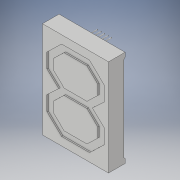
# Autodesk Inventor part: Digit
Saved by Autodesk Inventor 2019.3 (Build 233278000, 278)
## iProperties
Created: 2019-03-27
Part Number: Digit
Material: Generic
Document SubType Name: Modeling
Designer: Willist
Density: 1 g/cm^3
Appearance: Default
Author: Willist
Autodesk Inventor part; units mm, degrees
ref_plane "YZ Plane" through (0, 0, 0) normal (1, 0, 0) x (0, 1, 0)
ref_plane "XZ Plane" through (0, 0, 0) normal (0, 1, 0) x (-1, 0, 0)
ref_plane "XY Plane" through (0, 0, 0) normal (0, 0, 1) x (1, 0, 0)
sketch "Sketch1" plane through (0, 0, 0) normal (0, 0, 1) x (1, 0, 0)
  line L0 (-23.9, 34.85) -> (23.9, 34.85)
  line L1 (23.9, 34.85) -> (23.9, -34.85)
  line L2 (23.9, -34.85) -> (-23.9, -34.85)
  line L3 (-23.9, -34.85) -> (-23.9, 34.85)
  dimension "d0" = 47.8
  dimension "d1" = 69.7
  constraints: 8 end point, 2 parallel, 1 horizontal, 1 perpendicular
  measures "d0" distance of L1.end L2.end
  measures "d1" distance of L0.end L1.end
extrude "Extrusion1" add sketch "Sketch1" along normal blind 11
sketch "Sketch2" plane through (0, 0, 0) normal (0, 0, -1) x (-1, 0, 0)
  line L0 (-23.9, 34.85) -> (23.9, 34.85) projected
  line L1 (23.9, 34.85) -> (23.9, -34.85) projected
  line L2 (-23.9, 34.85) -> (23.9, 34.85)
  line L3 (23.9, 34.85) -> (23.9, 31.7132)
  line L4 (23.9, 31.7132) -> (-23.9, 31.7132)
  line L5 (-23.9, 31.7132) -> (-23.9, 34.85)
  line L6 (23.9, -34.85) -> (-23.9, -34.85) projected
  line L7 (-23.9, -34.85) -> (-23.9, 34.85) projected
  line L8 (23.9, -34.85) -> (-23.9, -34.85)
  line L9 (-23.9, -34.85) -> (-23.9, -31.7132)
  line L10 (-23.9, -31.7132) -> (23.9, -31.7132)
  line L11 (23.9, -31.7132) -> (23.9, -34.85)
  line L12 (-23.9, 34.85) -> (23.9, 34.85)
  line L13 (23.9, 34.85) -> (23.9, 31.7132)
  line L14 (23.9, 31.7132) -> (-23.9, 31.7132)
  line L15 (-23.9, 31.7132) -> (-23.9, 34.85)
  line L16 (-23.9, -31.7132) -> (23.9, -31.7132)
  line L17 (23.9, -31.7132) -> (23.9, -34.85)
  line L18 (23.9, -34.85) -> (-23.9, -34.85)
  line L19 (-23.9, -34.85) -> (-23.9, -31.7132)
  point P0 (0, 0)
  dimension "d4" = 3.1368
  dimension "d5" = 3.1368
  constraints: 32 end point, 8 parallel, 4 horizontal, 4 perpendicular, 2 point on line
  measures "d4" distance of L2.end L3.end
  measures "d5" distance of L8.end L9.end
extrude "Extrusion2" add sketch "Sketch2" along normal blind 1 contours L0 L1 L4 L5 | L10 L1 L6 L7
chamfer "Chamfer1" distance 1 distance2 1 1 edges at (0, 31.7132, 0) measured on face at (0, 31.2132, 0)
chamfer "Chamfer2" distance 1 distance2 1 1 edges at (0, -31.7132, 0) measured on face at (0, -31.2132, 0)
sketch "Sketch3" plane through (0, 0, 0) normal (0, 0, -1) x (-1, 0, 0)
  circle A0 centre (0, 30.1) radius 0.3
  circle A1 centre (2.54, 30.1) radius 0.3
  circle A2 centre (5.08, 30.1) radius 0.3
  line L0 (-23.9, 30.7132) -> (23.9, 30.7132) projected
  line L1 (0, 30.7132) -> (0, 27.4639)
  circle A3 centre (-2.54, 30.1) radius 0.3
  circle A4 centre (-5.08, 30.1) radius 0.3
  line L2 (-5.649, 0) -> (7.1976, 0)
  circle A5 centre (0, -30.1) radius 0.3
  circle A6 centre (2.54, -30.1) radius 0.3
  circle A7 centre (5.08, -30.1) radius 0.3
  circle A8 centre (-2.54, -30.1) radius 0.3
  circle A9 centre (-5.08, -30.1) radius 0.3
  point P0 (0, 0)
  dimension "d14" = 0.6
  dimension "d15" = 0.6
  dimension "d16" = 0.6
  constraints: 10 centre point, 7 symmetric about line, 4 end point, 1 horizontal, 1 midpoint, 1 vertical, 7 other
  measures "d14" diameter of A0
  measures "d15" diameter of A1
  measures "d16" diameter of A2
extrude "Extrusion3" add sketch "Sketch3" along normal blind 10
sketch "Sketch4" plane through (0, 0, 11) normal (0, 0, 1) x (1, 0, 0)
  line L0 (-28.3117, 29.0487) -> (26.925, 29.0487) construction
  line L1 (26.925, 29.0487) -> (26.925, -28.8882) construction
  line L2 (26.925, -28.8882) -> (-28.3117, -28.8882) construction
  line L3 (-28.3117, -28.8882) -> (-28.3117, 29.0487) construction
  line L4 (20.8139, -18.7031) -> (10.2024, -28.8882)
  line L5 (10.2024, -28.8882) -> (-10.0732, -28.8882)
  line L6 (-10.0732, -28.8882) -> (-20.6373, -18.7031)
  line L7 (-20.6373, -18.7031) -> (-20.6373, -7.9494)
  line L8 (-20.6373, -7.9494) -> (-12.0628, 0.0566)
  line L9 (-12.0628, 0.0566) -> (-20.6373, 8.0626)
  line L10 (-20.6373, 8.0626) -> (-20.6373, 18.7688)
  line L11 (-20.6373, 18.7688) -> (-10.0732, 29.0487)
  line L12 (-10.0732, 29.0487) -> (10.155, 29.0487)
  line L13 (10.155, 29.0487) -> (20.8139, 18.7688)
  line L14 (20.8139, 18.7688) -> (20.8139, 8.0626)
  line L15 (20.8139, 8.0626) -> (12.192, 0.0566)
  line L16 (12.192, 0.0566) -> (20.8139, -7.9968)
  line L17 (20.8139, -7.9968) -> (20.8139, -18.7031)
  line L18 (16.124, -16.9029) -> (16.124, -9.797)
  line L19 (16.124, -9.797) -> (8.3075, -2.2173)
  line L20 (8.3075, -2.2173) -> (-8.2256, -2.2173)
  line L21 (-8.2256, -2.2173) -> (-15.9948, -9.7496)
  line L22 (-15.9948, -9.7496) -> (-15.9948, -16.9029)
  line L23 (-15.9948, -16.9029) -> (-8.2256, -24.4352)
  line L24 (-8.2256, -24.4352) -> (8.3075, -24.4352)
  line L25 (8.3075, -24.4352) -> (16.124, -16.9029)
  line L26 (16.124, 9.8627) -> (16.124, 16.9687)
  line L27 (16.124, 16.9687) -> (8.3075, 24.5483)
  line L28 (8.3075, 24.5483) -> (-8.2256, 24.5483)
  line L29 (-8.2256, 24.5483) -> (-15.9948, 17.016)
  line L30 (-15.9948, 17.016) -> (-15.9948, 9.8627)
  line L31 (-15.9948, 9.8627) -> (-8.2256, 2.3305)
  line L32 (-8.2256, 2.3305) -> (8.3075, 2.3305)
  line L33 (8.3075, 2.3305) -> (16.124, 9.8627)
  point P0 (0, 0)
  constraints: 2 other
extrude "Extrusion4" cut sketch "Sketch4" against normal blind 1
body "Solid1"
